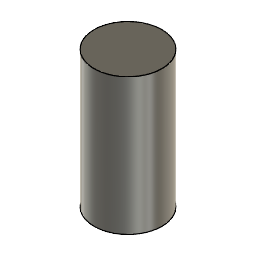
peg (Autodesk Fusion 360 design; units mm, degrees)
Autodesk Fusion 360 part; units mm, degrees
sketch "Sketch1" plane through (0, 0, 0) normal (0, 0, 1) x (1, 0, 0)
  circle A0 centre (0, 0) radius 4.95
  dimension "d1" = 9.9
  constraint coincident A0.centre origin
  measures "d1" diameter of A0
extrude "Extrude1" add sketch "Sketch1" along normal blind 9.8
extrude "Extrude2" add 1 faces at (1.6316, -1.613, 9.8) along direction (0, 0, 1) blind 1.5
extrude "Extrude3" cut 1 faces at (1.6316, -1.613, 11.3) along direction (0, 0, -1) blind 1.3
extrude "Extrude4" cut 1 faces at (1.6316, -1.613, 10) along direction (0, 0, -1) blind 0.05
extrude "Extrude5" cut 1 faces at (1.6316, -1.613, 9.95) along direction (0, 0, -1) blind 16
sketch "Sketch2" plane through (0, 0, 0) normal (0, 0, 1) x (1, 0, 0)
  circle A0 centre (0, 0) radius 2.4625
  dimension "d12" = 4.925
  constraint coincident A0.centre origin
  measures "d12" diameter of A0
extrude "Extrude6" add sketch "Sketch2" along normal blind 9.925
